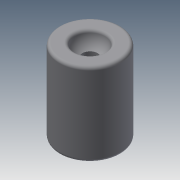
# Autodesk Inventor part: valecky_na_otocny_kruh
Saved by Autodesk Inventor 2013 (Build 170138000, 138)
## iProperties
Created: 2013-06-08
Part Number: valecky_na_otocny_kruh
Material: Generic
Document SubType Name: Modeling
Designer: idle-rug
Density: 1 g/cm^3
Author: idle-rug
Autodesk Inventor part; units mm, degrees
ref_plane "YZ Plane" through (0, 0, 0) normal (1, 0, 0) x (0, 1, 0)
ref_plane "XZ Plane" through (0, 0, 0) normal (0, 1, 0) x (-1, 0, 0)
ref_plane "XY Plane" through (0, 0, 0) normal (0, 0, 1) x (1, 0, 0)
sketch "Sketch1" plane through (0, 0, 0) normal (0, 0, 1) x (1, 0, 0)
  circle A0 centre (0, 0) radius 5
  dimension "d0" = 10
  constraints: 1 centre point, 1 coincident
  measures "d0" diameter of A0
extrude "Extrusion1" add sketch "Sketch1" along normal blind 13.5
sketch "Sketch2" plane through (0, 0, 13.5) normal (0, 0, 1) x (1, 0, 0)
  circle A0 centre (0, 0) radius 5 projected
  circle A1 centre (0, 0) radius 1.25
  dimension "d3" = 2.5
  constraints: 1 centre point, 1 coincident
  measures "d3" diameter of A1
extrude "Extrusion2" cut sketch "Sketch2" against normal blind 13.5 contours A1
sketch "Sketch4" plane through (0, 0, 13.5) normal (0, 0, 1) x (1, 0, 0)
  circle A0 centre (0, 0) radius 5 projected
  circle A1 centre (0, 0) radius 2.5
  line L0 (-1.5, -2) -> (1.5, 2)
  dimension "d6" = 5
  constraints: 2 end point, 2 point on circle, 1 centre point, 1 coincident, 1 midpoint
  measures "d6" diameter of A1
revolve "Revolution1" cut sketch "Sketch4" angle 360 about axis through (-1.5, -2, 13.5) along (0.6, 0.8, 0) picked at (0.5015, -1.2253) contours A1 L0
sketch "Sketch6" plane through (0, 0, 0) normal (0, 0, -1) x (-1, 0, 0)
  circle A0 centre (0, 0) radius 5 projected
  circle A1 centre (0, 0) radius 2.5
  line L0 (-1.0028, -2.29) -> (1.0028, 2.29)
  dimension "d8" = 5
  constraints: 2 end point, 2 point on circle, 1 centre point, 1 coincident, 1 midpoint
  measures "d8" diameter of A1
revolve "Revolution2" cut sketch "Sketch6" angle 360 about axis through (1.0028, -2.29, 0) along (-0.4011329, 0.9160199, 0) picked at (0.733, -0.3965) contours A1 L0
fillet "Fillet1" radius 0.5 6 edges at (-5, 0, 13.5) (2, -1.5, 13.5) (-2, 1.5, 13.5) (-5, 0, 0) (2.29, 1.0028, 0) (-2.29, -1.0028, 0)
body "Solid1"
